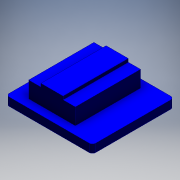
# Autodesk Inventor part: chamberInsertFlat
Saved by Autodesk Inventor 2016 (Build 200138000, 138)
## iProperties
Created: 2016-10-05
Part Number: chamberInsertFlat
Material: Generic
Document SubType Name: Modeling
Designer: sims01
Density: 1 g/cm^3
Appearance: Default
Author: sims01
Autodesk Inventor part; units mm, degrees
ref_plane "YZ Plane" through (0, 0, 0) normal (1, 0, 0) x (0, 1, 0)
ref_plane "XZ Plane" through (0, 0, 0) normal (0, 1, 0) x (-1, 0, 0)
ref_plane "XY Plane" through (0, 0, 0) normal (0, 0, 1) x (1, 0, 0)
sketch "Sketch1" plane through (0, 0, 0) normal (0, 0, 1) x (1, 0, 0)
  line L0 (-24.5, 25) -> (24.5, 25)
  line L1 (26.5, 23) -> (26.5, -23)
  line L2 (24.5, -25) -> (-24.5, -25)
  line L3 (-26.5, -23) -> (-26.5, 23)
  arc A0 (-24.5, 25) -> (-26.5, 23) centre (-24.5, 23) ccw
  arc A1 (-26.5, -23) -> (-24.5, -25) centre (-24.5, -23) ccw
  arc A2 (24.5, -25) -> (26.5, -23) centre (24.5, -23) ccw
  arc A3 (26.5, 23) -> (24.5, 25) centre (24.5, 23) ccw
  point P0 (0, 0)
  point P1 (-26.5, 25)
  point P2 (26.5, -25)
  point P3 (26.5, 25)
  dimension "d0" = 53
  dimension "d2" = 2
  dimension "d3" = 25
  dimension "d4" = 50
  dimension "d5" = 26.5
  constraints: 8 end point, 8 point on circle, 8 tangent, 6 point on line, 4 centre point, 3 equal radius, 2 parallel, 1 horizontal, 1 perpendicular
  measures "d0" distance of point (-26.5, 25) point (26.5, 25)
  measures "d2" radius of A0
  measures "d3" distance from line of point (0, 0) L0
  measures "d4" distance between parallel lines of L2 L0
  measures "d5" distance from line of point (0, 0) L1
extrude "base" add sketch "Sketch1" along normal blind 5
sketch "Sketch3" plane through (0, 0, 0) normal (0, 0, -1) x (-1, 0, 0)
  line L0 (26.5, 23) -> (26.5, -23) projected
  circle A0 centre (-3.5, 15) radius 2.825
  circle A1 centre (-18.5, 0) radius 2.825
  circle A2 centre (-3.5, 0) radius 2.825
  circle A3 centre (-3.5, -15) radius 2.825
  circle A4 centre (11.5, 0) radius 2.825
  point P0 (0, 0)
  dimension "d14" = 15
  dimension "d15" = 15
  dimension "d16" = 15
  dimension "d17" = 15
  dimension "d18" = 15
  dimension "d56" = 5.65
  dimension "d57" = 5.65
  dimension "d58" = 5.65
  dimension "d59" = 5.65
  dimension "d60" = 5.65
  constraints: 5 centre point, 5 coincident, 3 horizontal alignment, 2 vertical alignment
  measures "d14" distance from line of L0 point (11.5, 0)
  measures "d15" distance of point (-3.5, 0) point (11.5, 0)
  measures "d16" distance of point (-18.5, 0) point (-3.5, 0)
  measures "d17" distance of point (-3.5, -15) point (-3.5, 0)
  measures "d18" distance of point (-3.5, 15) point (-3.5, 0)
  measures "d56" diameter of A0
  measures "d57" diameter of A1
  measures "d58" diameter of A2
  measures "d59" diameter of A3
  measures "d60" diameter of A4
extrude "magnetExt" cut sketch "Sketch3" against normal blind 2.5
sketch "Sketch7" plane through (0, 0, 5) normal (0, 0, 1) x (1, 0, 0)
  line L0 (-17.6, 20) -> (11, 20)
  line L1 (11, 20) -> (11, -20)
  line L2 (11, -20) -> (-17.6, -20)
  line L3 (-17.6, -20) -> (-17.6, 20)
  line L4 (-26.5, 23) -> (-26.5, -23) projected
  point P0 (0, 0)
  dimension "d70" = 40
  dimension "d71" = 20
  dimension "d72" = 28.6
  dimension "d73" = 8.9
  constraints: 8 end point, 2 parallel, 1 horizontal, 1 perpendicular
  measures "d70" distance of L2.end L0.start
  measures "d71" distance from line of point (0, 0) L0
  measures "d72" distance of L0.start L0.end
  measures "d73" distance between parallel lines of L4 L3
extrude "spacerOne" add sketch "Sketch7" along normal blind 10
sketch "Sketch8" plane through (0, 0, 15) normal (0, 0, 1) x (1, 0, 0)
  line L0 (-10.1, 20) -> (3.5, 20)
  line L1 (3.5, 20) -> (3.5, -20)
  line L2 (3.5, -20) -> (-10.1, -20)
  line L3 (-10.1, -20) -> (-10.1, 20)
  line L4 (-26.5, 23) -> (-26.5, -23) projected
  point P0 (0, 0)
  dimension "d76" = 40
  dimension "d77" = 20
  dimension "d78" = 13.6
  dimension "d79" = 30
  constraints: 8 end point, 2 parallel, 1 horizontal, 1 perpendicular
  measures "d76" distance of L0.end L1.end
  measures "d77" distance from line of point (0, 0) L0
  measures "d78" distance between parallel lines of L1 L3
  measures "d79" distance between parallel lines of L4 L1
extrude "sample" add sketch "Sketch8" along normal blind 2
equation "\"d3\" = 0.5 * d4"
equation "\"d5\" = 0.5 * d0"
equation "\"d16\" = d15"
equation "\"d17\" = d15"
equation "\"d18\" = d15"
equation "\"d56\" = d60"
equation "\"d57\" = d60"
equation "\"d58\" = d60"
equation "\"d59\" = d60"
equation "\"d71\" = 0.5 * d70"
equation "\"d77\" = 0.5 * d76"
equation "\"d1\" = d0"
body "Solid1"
